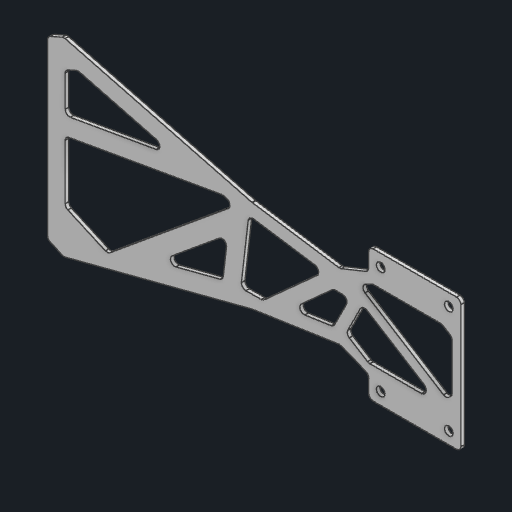
# Autodesk Inventor part: ShoulderMount
Saved by Autodesk Inventor 2023 (Build 270158000, 158)
## iProperties
Created: 2024-03-14
Part Number: ShoulderMount
Material: Generic
Document SubType Name: Sheet Metal
Designer: LattePanda
Density: 1 g/cm^3
Sheet Metal Rule: Default
Appearance: Default
Author: LattePanda
Autodesk Inventor part; units mm, degrees
ref_plane "YZ Plane" through (0, 0, 0) normal (1, 0, 0) x (0, 1, 0)
ref_plane "XZ Plane" through (0, 0, 0) normal (0, 1, 0) x (-1, 0, 0)
ref_plane "XY Plane" through (0, 0, 0) normal (0, 0, 1) x (1, 0, 0)
sketch "Mount" plane through (0, 0, 0) normal (0, 0, 1) x (1, 0, 0)
  circle A0 centre (-15.5, -1.5) radius 1.621 construction
  circle A1 centre (15.5, -1.5) radius 1.621 construction
  circle A2 centre (-15.5, -50.5) radius 1.621 construction
  circle A3 centre (15.5, -50.5) radius 1.621 construction
  line L0 (19, 6) -> (-19, 6) construction
  line L1 (19, -58) -> (-19, -58) construction
  circle A4 centre (-15.5, -1.5) radius 2
  circle A5 centre (15.5, -1.5) radius 2
  circle A6 centre (-15.5, -50.5) radius 2
  circle A7 centre (15.5, -50.5) radius 2
  line L2 (-21, 4) -> (21, 4)
  line L3 (21, 4) -> (21, -56)
  line L4 (21, -56) -> (-21, -56)
  line L5 (-21, -56) -> (-21, -46.5047)
  line L6 (21, -51.5858) -> (21, -0.4142) construction
  line L7 (-21, 6) -> (-21, -6) construction
  line L8 (-19, -6) -> (19, -6) construction
  line L9 (-19, -46) -> (19, -46) construction
  line L10 (11.0973, -13.4202) -> (13.4116, -6.5798) construction
  line L11 (-17, -43.4537) -> (-13.9151, -46) construction
  line L12 (-21, -6) -> (-34, -11.2523)
  line L13 (-21, -26.2523) -> (-34, -26.2523) construction
  line L14 (-34, -26.2523) -> (-34, -11.2523) construction
  line L15 (-21, -46.5047) -> (-34, -41.2523)
  line L16 (-34, -26.2523) -> (-34, -41.2523) construction
  line L17 (-74, -47.2523) -> (-74, -5.2523) construction
  line L18 (-74, -5.2523) -> (-159.8345, 16.9952)
  line L19 (-159.8345, 16.9952) -> (-167.1457, 13.7477)
  line L20 (-167.1457, 13.7477) -> (-167.1457, -26.2523)
  line L21 (-167.1457, -26.2523) -> (-74, -26.2523) construction
  line L22 (-74, -47.2523) -> (-159.8345, -69.4998)
  line L23 (-159.8345, -69.4998) -> (-167.1457, -66.2523)
  line L24 (-167.1457, -66.2523) -> (-167.1457, -26.2523)
  line L25 (-34, -11.2523) -> (-74, -5.2523)
  line L26 (-34, -41.2523) -> (-74, -47.2523)
  line L27 (-74, -47.2523) -> (-34, -11.2523) construction
  line L28 (-34, -11.2523) -> (21, -45.6202) construction
  line L29 (-41.1721, -16.2437) -> (-75.5743, -11.0833)
  line L30 (-56.6745, -38.5864) -> (-37, -20.8793)
  line L31 (-37, -20.8793) -> (-37, -35.6352)
  line L32 (-37, -35.6352) -> (-56.6745, -38.5864)
  line L33 (-37, -20.8793) -> (-41.1721, -16.2437) construction
  line L34 (-75.5743, -11.0833) -> (-79.1803, -41.4923)
  line L35 (-79.1803, -41.4923) -> (-69.0783, -41.3593)
  line L36 (-69.0783, -41.3593) -> (-41.1721, -16.2437)
  line L37 (-21, -6) -> (-21, 4)
  line L38 (-21, -46.5047) -> (-21, -6) construction
  line L39 (-37, -35.6352) -> (-29.5556, -20.8793)
  line L40 (-29.5556, -20.8793) -> (-37, -20.8793)
  line L41 (-31.3485, -35.5336) -> (-23.7162, -20.4052)
  line L42 (-23.7162, -20.4052) -> (6.0353, -38.996)
  line L43 (6.0353, -38.996) -> (4.1582, -42)
  line L44 (4.1582, -42) -> (-21, -42)
  line L45 (-21, -42) -> (-31.3485, -35.5336)
  line L46 (14.4436, -38.3543) -> (17, -35.8395)
  line L47 (17, -35.8395) -> (17, -12.9233)
  line L48 (17, -12.9233) -> (12.2545, -10)
  line L49 (12.2545, -10) -> (-19.2449, -10)
  line L50 (-19.2449, -10) -> (-25.6209, -13.3192)
  line L51 (-25.6209, -13.3192) -> (14.4436, -38.3543)
  line L52 (-81.7814, -10.4668) -> (-87.5894, -8.9614)
  line L53 (-81.7814, -10.4668) -> (-139.7038, -58.2144)
  line L54 (-87.3497, -42.4481) -> (-117.4718, -50.2555)
  line L55 (-117.4718, -50.2555) -> (-85.1123, -23.5803)
  line L56 (-85.1123, -23.5803) -> (-87.3497, -42.4481)
  line L57 (-87.5894, -8.9614) -> (-159.1457, -21.5787)
  line L58 (-159.1457, -21.5787) -> (-159.1457, -49.5787)
  line L59 (-159.1457, -49.5787) -> (-139.7038, -58.2144)
  line L60 (-159.1457, -13.4553) -> (-108.6138, -4.5451)
  line L61 (-108.6138, -4.5451) -> (-153.4481, 7.0755)
  line L62 (-153.4481, 7.0755) -> (-159.1457, 4.5447)
  line L63 (-159.1457, 4.5447) -> (-159.1457, -13.4553)
  point P0 (0, 0)
  point P1 (-5.5886, -25.8367)
  dimension "d0" = 4
  dimension "d1" = 4
  dimension "d2" = 4
  dimension "d3" = 4
  dimension "d7" = 2
  dimension "d8" = 2
  dimension "d15" = 80
  dimension "d16" = 8
  dimension "d17" = 13
  dimension "d18" = 40
  dimension "d19" = 93.1457
  dimension "d20" = 30
  dimension "d21" = 42
  dimension "d24" = 6
  dimension "d26" = 6
  dimension "d30" = 3
  dimension "d31" = 32
  dimension "d33" = 112
  dimension "d34" = 174
  dimension "d35" = 80
  dimension "d36" = 5
  dimension "d37" = 5.5
  dimension "d38" = 8
  dimension "d39" = 8
  dimension "d40" = 8
  dimension "d41" = 8
  dimension "d42" = 7
  dimension "d43" = 8
  dimension "d44" = 8
  dimension "d45" = 50.5
  dimension "d46" = 28
  dimension "d47" = 18
  dimension "d48" = 6
  dimension "d49" = 19
  dimension "d51" = 5
  dimension "d52" = 4
  dimension "d53" = 4
  dimension "d54" = 4
  dimension "d55" = 41.25
  measures "d0" diameter of A4
  measures "d1" diameter of A5
  measures "d2" diameter of A6
  measures "d3" diameter of A7
  measures "d8" distance between parallel lines of L1 L4
  measures "d15" distance of L24.start L19.end
  measures "d16" distance of L18.end L19.end
  measures "d17" distance between parallel lines of L5 L14
  measures "d18" distance between parallel lines of L14 L17
  measures "d19" distance between parallel lines of L17 L20
  measures "d20" distance of L15.end L12.end
  measures "d21" distance of L17.start L17.end
  measures "d24" distance between parallel lines of L25 L29
  measures "d26" distance between parallel lines of L26 L32
  measures "d30" distance between parallel lines of L14 L31
  measures "d31" angle of L8 L28
  measures "d33" angle of L7 L12
  measures "d34" angle of L25 L18
  measures "d35" angle of L20 L57
  measures "d36" distance between parallel lines of L41 L39
  measures "d37" angle of L12 L50
  measures "d38" distance between parallel lines of L18 L61
  measures "d39" distance between parallel lines of L57 L60
  measures "d40" distance between parallel lines of L20 L63
  measures "d41" distance between parallel lines of L55 L53
  measures "d42" distance between parallel lines of L18 L52
  measures "d43" distance between parallel lines of L34 L56
  measures "d44" distance between parallel lines of L22 L54
  measures "d45" angle of L53 L24
  measures "d46" distance of L57.end L58.end
  measures "d47" distance of L62.end L60.start
  measures "d48" distance of L52.start L52.end
  measures "d49" distance of L55.end L54.start
  measures "d51" distance from line of point (-5.589, -25.837) L42
  measures "d52" distance between parallel lines of L3 L47
  measures "d53" distance between parallel lines of L8 L49
  measures "d54" distance between parallel lines of L9 L44
  measures "d55" angle of L36 L34
extrude "Plate1" add sketch "Mount" along normal blind 1.6002
fillet "MountFilletsFeature" radius 2 46 edges at (21, 4, 0.8001) (-21, 4, 0.8001) (21, -56, 0.8001) (-21, -56, 0.8001) (-21, -6, 0.8001) (-34, -11.2523, 0.8001) (-74, -5.2523, 0.8001) (-21, -46.5047, 0.8001) (-159.8345, 16.9952, 0.8001) (-34, -41.2523, 0.8001) (-167.1457, 13.7477, 0.8001) (-74, -47.2523, 0.8001) (-167.1457, -26.2523, 0.8001) (-159.8345, -69.4998, 0.8001) (-167.1457, -66.2523, 0.8001) (-139.7038, -58.2144, 0.8001) (-81.7814, -10.4668, 0.8001) (-87.5894, -8.9614, 0.8001) (-159.1457, -21.5787, 0.8001) (-159.1457, -49.5787, 0.8001) (-85.1123, -23.5803, 0.8001) (-87.3497, -42.4481, 0.8001) (-117.4718, -50.2555, 0.8001) (-79.1803, -41.4923, 0.8001) (-75.5743, -11.0833, 0.8001) (-69.0783, -41.3593, 0.8001) (-41.1721, -16.2437, 0.8001) (-29.5556, -20.8793, 0.8001) (-37, -20.8793, 0.8001) (-56.6745, -38.5864, 0.8001) (-37, -35.6352, 0.8001) (-21, -42, 0.8001) (-31.3485, -35.5336, 0.8001) (4.1582, -42, 0.8001) (6.0353, -38.996, 0.8001) (-23.7162, -20.4052, 0.8001) (-159.1457, 4.5447, 0.8001) (-159.1457, -13.4553, 0.8001) (-108.6138, -4.5451, 0.8001) (-153.4481, 7.0755, 0.8001) (-25.6209, -13.3192, 0.8001) (14.4436, -38.3543, 0.8001) (17, -35.8395, 0.8001) (17, -12.9233, 0.8001) (12.2545, -10, 0.8001) (-19.2449, -10, 0.8001)
fillet_without_effect "Fillet2"
equation "\"d24\" = d22"
equation "\"d26\" = d22"
equation "\"d30\" = 0.5 * d22"
equation "\"d9\" = Thickness"
equation "\"BendRadius\" = Thickness"
equation "\"BendReliefWidth\" = Thickness"
equation "\"BendReliefDepth\" = 0.5 * Thickness"
equation "\"CornerReliefSize\" = 4 * Thickness"
equation "\"MinimumRemnant\" = 2 * Thickness"
equation "\"TransitionRadius\" = BendRadius"
equation "\"JacobiRadiusSize\" = BendRadius"
equation "\"GapSize\" = Thickness"
equation "\"d22\" = 6"
equation "\"Thickness\" = 1.6002"
body "Solid1"
